Autodesk Fusion 360 part; units mm, degrees
note: some values were not read from the file. Set by a fixed rule: which face or edge a step refers to.
(part 2 of 2)
  arc A109 (-60.8901, 219.4175) -> (-60.8901, 225.0825) centre (-63.7145, 222.25) ccw construction
  line L110 (-63.3611, 192.0464) -> (-60.8901, 189.5825) construction
  arc A110 (-60.8901, 183.9175) -> (-60.8901, 189.5825) centre (-63.7145, 186.75) ccw construction
  line L111 (-60.8901, 183.9175) -> (-63.3611, 181.4536) construction
  arc A111 (-70.1855, 184.2861) -> (-63.3611, 181.4536) centre (-66.1855, 184.2861) ccw construction
  line L112 (-70.1855, 184.2861) -> (-70.1855, 189.2139) construction
  arc A112 (-63.3611, 192.0464) -> (-70.1855, 189.2139) centre (-66.1855, 189.2139) ccw construction
  line L113 (-60.8901, 148.4175) -> (-63.3611, 145.9536) construction
  arc A113 (-70.1855, 148.7861) -> (-63.3611, 145.9536) centre (-66.1855, 148.7861) ccw construction
  line L114 (-70.1855, 148.7861) -> (-70.1855, 153.7139) construction
  arc A114 (-63.3611, 156.5464) -> (-70.1855, 153.7139) centre (-66.1855, 153.7139) ccw construction
  line L115 (-63.3611, 156.5464) -> (-60.8901, 154.0825) construction
  arc A115 (-60.8901, 148.4175) -> (-60.8901, 154.0825) centre (-63.7145, 151.25) ccw construction
  line L116 (-63.3611, 121.0464) -> (-60.8901, 118.5825) construction
  arc A116 (-60.8901, 112.9175) -> (-60.8901, 118.5825) centre (-63.7145, 115.75) ccw construction
  line L117 (-60.8901, 112.9175) -> (-63.3611, 110.4536) construction
  arc A117 (-70.1855, 113.2861) -> (-63.3611, 110.4536) centre (-66.1855, 113.2861) ccw construction
  line L118 (-70.1855, 113.2861) -> (-70.1855, 118.2139) construction
  arc A118 (-63.3611, 121.0464) -> (-70.1855, 118.2139) centre (-66.1855, 118.2139) ccw construction
  line L119 (-55.2089, 159.715) -> (-61.6799, 166.1675) construction
  arc A119 (-61.6799, 171.8325) -> (-61.6799, 166.1675) centre (-58.8555, 169) ccw construction
  line L120 (-61.6799, 171.8325) -> (-55.2089, 178.285) construction
  arc A120 (-49.5601, 178.285) -> (-55.2089, 178.285) centre (-52.3845, 175.4525) ccw construction
  line L121 (-49.5601, 178.285) -> (-43.0891, 171.8325) construction
  arc A121 (-43.0891, 166.1675) -> (-43.0891, 171.8325) centre (-45.9135, 169) ccw construction
  line L122 (-43.0891, 166.1675) -> (-49.5601, 159.715) construction
  arc A122 (-55.2089, 159.715) -> (-49.5601, 159.715) centre (-52.3845, 162.5475) ccw construction
  circle A123 centre (-52.3845, 115.75) radius 3 construction
  line L123 (-49.5601, 213.785) -> (-43.0891, 207.3325) construction
  arc A124 (-43.0891, 201.6675) -> (-43.0891, 207.3325) centre (-45.9135, 204.5) ccw construction
  line L124 (-43.0891, 201.6675) -> (-49.5601, 195.215) construction
  arc A125 (-55.2089, 195.215) -> (-49.5601, 195.215) centre (-52.3845, 198.0475) ccw construction
  line L125 (-55.2089, 195.215) -> (-61.6799, 201.6675) construction
  arc A126 (-61.6799, 207.3325) -> (-61.6799, 201.6675) centre (-58.8555, 204.5) ccw construction
  line L126 (-61.6799, 207.3325) -> (-55.2089, 213.785) construction
  arc A127 (-49.5601, 213.785) -> (-55.2089, 213.785) centre (-52.3845, 210.9525) ccw construction
  line L127 (-49.5601, 142.785) -> (-43.0891, 136.3325) construction
  arc A128 (-43.0891, 130.6675) -> (-43.0891, 136.3325) centre (-45.9135, 133.5) ccw construction
  line L128 (-43.0891, 130.6675) -> (-49.5601, 124.215) construction
  arc A129 (-55.2089, 124.215) -> (-49.5601, 124.215) centre (-52.3845, 127.0475) ccw construction
  line L129 (-55.2089, 124.215) -> (-61.6799, 130.6675) construction
  arc A130 (-61.6799, 136.3325) -> (-61.6799, 130.6675) centre (-58.8555, 133.5) ccw construction
  line L130 (-61.6799, 136.3325) -> (-55.2089, 142.785) construction
  arc A131 (-49.5601, 142.785) -> (-55.2089, 142.785) centre (-52.3845, 139.9525) ccw construction
  circle A132 centre (-52.3845, 222.25) radius 3 construction
  circle A133 centre (-52.3845, 151.25) radius 3 construction
  circle A134 centre (-52.3845, 186.75) radius 3 construction
  line L131 (-57.6684, 104.8325) -> (-55.2089, 107.285) construction
  arc A135 (-49.5601, 107.285) -> (-55.2089, 107.285) centre (-52.3845, 104.4525) ccw construction
  line L132 (-49.5601, 107.285) -> (-47.1006, 104.8325) construction
  arc A136 (-49.925, 98) -> (-47.1006, 104.8325) centre (-49.925, 102) ccw construction
  line L133 (-49.925, 98) -> (-54.844, 98) construction
  arc A137 (-57.6684, 104.8325) -> (-54.844, 98) centre (-54.844, 102) ccw construction
  line L134 (-52.3845, 151.25) -> (52.3845, 151.25) construction
  circle A138 centre (-10, 151.25) radius 3.5
  circle A139 centre (10, 151.25) radius 3.5
  line L135 (0, 222.25) -> (0, 115.75) construction
  dimension "d99" = 7
  dimension "d100" = 20
  constraint coincident A133.centre L134.start
  constraint coincident A48.centre L134.end
  constraint coincident L134 A138.centre
  constraint coincident L134 A139.centre
  constraint coincident A90.centre L135.start
  constraint coincident A91.centre L135.end
  constraint equal A138 A139
  constraint symmetric A138 A139 L135
  measures "d99" diameter of A138
  measures "d100" distance of A138.centre A139.centre
extrude "Extrude12" cut sketch "Sketch13" against normal up to surface (18 mm away) contours L56 A52 L57 A139 | L56 A52 L57 A139 | L74 L76 A72 A138 | L74 L76 A72 A138
extrude "Extrude13" add sketch "Sketch13" against normal up to surface (18 mm away) contours L56 L57 A53 L58 A54 A139 | L74 A70 L75 A71 L76 A138 | A84
sketch "Sketch14" plane through (174.5, 0, 0) normal (1, 0, 0) x (0, 0, -1)
  circle A0 centre (-26.5204, 133.5) radius 7.5
  circle A1 centre (26.5204, 204.5) radius 7.5
  circle A2 centre (-26.5204, 169) radius 7.5
  circle A3 centre (26.5204, 133.5) radius 7.5
  circle A4 centre (26.5204, 169) radius 7.5
  circle A5 centre (-26.5204, 204.5) radius 7.5
  line L0 (-70.1855, 184.2861) -> (-70.1855, 189.2139)
  arc A6 (-63.3611, 192.0464) -> (-70.1855, 189.2139) centre (-66.1855, 189.2139) ccw
  line L1 (-63.3611, 192.0464) -> (-60.8901, 189.5825)
  arc A7 (-60.8901, 183.9175) -> (-60.8901, 189.5825) centre (-63.7145, 186.75) ccw
  line L2 (-60.8901, 183.9175) -> (-63.3611, 181.4536)
  arc A8 (-70.1855, 184.2861) -> (-63.3611, 181.4536) centre (-66.1855, 184.2861) ccw
  line L3 (-70.1855, 219.7861) -> (-70.1855, 224.7139)
  arc A9 (-63.3611, 227.5464) -> (-70.1855, 224.7139) centre (-66.1855, 224.7139) ccw
  line L4 (-63.3611, 227.5464) -> (-60.8901, 225.0825)
  arc A10 (-60.8901, 219.4175) -> (-60.8901, 225.0825) centre (-63.7145, 222.25) ccw
  line L5 (-60.8901, 219.4175) -> (-63.3611, 216.9536)
  arc A11 (-70.1855, 219.7861) -> (-63.3611, 216.9536) centre (-66.1855, 219.7861) ccw
  line L6 (-64.5205, 240) -> (-83, 240)
  line L7 (-83, 240) -> (-83, 116)
  line L8 (-83, 116) -> (-92, 107)
  line L9 (-92, 107) -> (-92, 90)
  line L10 (-92, 90) -> (92, 90)
  line L11 (92, 90) -> (92, 107)
  line L12 (92, 107) -> (83, 116)
  line L13 (83, 116) -> (83, 240)
  line L14 (83, 240) -> (64.5205, 240)
  line L15 (64.5205, 240) -> (55.2089, 230.715)
  arc A12 (49.5601, 230.715) -> (55.2089, 230.715) centre (52.3845, 233.5475) ccw
  line L16 (49.5601, 230.715) -> (40.2485, 240)
  line L17 (40.2485, 240) -> (12.7923, 240)
  line L18 (12.7923, 240) -> (2.7628, 230.4203)
  arc A13 (-2.7628, 230.4203) -> (2.7628, 230.4203) centre (0, 233.3129) ccw
  line L19 (-2.7628, 230.4203) -> (-12.7923, 240)
  line L20 (-12.7923, 240) -> (-40.2485, 240)
  line L21 (-40.2485, 240) -> (-49.5601, 230.715)
  arc A14 (-55.2089, 230.715) -> (-49.5601, 230.715) centre (-52.3845, 233.5475) ccw
  line L22 (-55.2089, 230.715) -> (-64.5205, 240)
  line L23 (-34.5835, 224.7139) -> (-34.5835, 219.7861)
  arc A15 (-41.4079, 216.9536) -> (-34.5835, 219.7861) centre (-38.5835, 219.7861) ccw
  line L24 (-41.4079, 216.9536) -> (-43.8789, 219.4175)
  arc A16 (-43.8789, 225.0825) -> (-43.8789, 219.4175) centre (-41.0545, 222.25) ccw
  line L25 (-43.8789, 225.0825) -> (-41.4079, 227.5464)
  arc A17 (-34.5835, 224.7139) -> (-41.4079, 227.5464) centre (-38.5835, 224.7139) ccw
  line L26 (-34.5835, 189.2139) -> (-34.5835, 184.2861)
  arc A18 (-41.4079, 181.4536) -> (-34.5835, 184.2861) centre (-38.5835, 184.2861) ccw
  line L27 (-41.4079, 181.4536) -> (-43.8789, 183.9175)
  arc A19 (-43.8789, 189.5825) -> (-43.8789, 183.9175) centre (-41.0545, 186.75) ccw
  line L28 (-43.8789, 189.5825) -> (-41.4079, 192.0464)
  arc A20 (-34.5835, 189.2139) -> (-41.4079, 192.0464) centre (-38.5835, 189.2139) ccw
  line L29 (-34.5835, 153.7139) -> (-34.5835, 148.7861)
  arc A21 (-41.4079, 145.9536) -> (-34.5835, 148.7861) centre (-38.5835, 148.7861) ccw
  line L30 (-41.4079, 145.9536) -> (-43.8789, 148.4175)
  arc A22 (-43.8789, 154.0825) -> (-43.8789, 148.4175) centre (-41.0545, 151.25) ccw
  line L31 (-43.8789, 154.0825) -> (-41.4079, 156.5464)
  arc A23 (-34.5835, 153.7139) -> (-41.4079, 156.5464) centre (-38.5835, 153.7139) ccw
  line L32 (-34.5835, 118.2139) -> (-34.5835, 113.2861)
  arc A24 (-41.4079, 110.4536) -> (-34.5835, 113.2861) centre (-38.5835, 113.2861) ccw
  line L33 (-41.4079, 110.4536) -> (-43.8789, 112.9175)
  arc A25 (-43.8789, 118.5825) -> (-43.8789, 112.9175) centre (-41.0545, 115.75) ccw
  line L34 (-43.8789, 118.5825) -> (-41.4079, 121.0464)
  arc A26 (-34.5835, 118.2139) -> (-41.4079, 121.0464) centre (-38.5835, 118.2139) ccw
  line L35 (-49.925, 98) -> (-54.844, 98)
  arc A27 (-57.6684, 104.8325) -> (-54.844, 98) centre (-54.844, 102) ccw
  line L36 (-57.6684, 104.8325) -> (-55.2089, 107.285)
  arc A28 (-49.5601, 107.285) -> (-55.2089, 107.285) centre (-52.3845, 104.4525) ccw
  line L37 (-49.5601, 107.285) -> (-47.1006, 104.8325)
  arc A29 (-49.925, 98) -> (-47.1006, 104.8325) centre (-49.925, 102) ccw
  line L38 (-70.1855, 113.2861) -> (-70.1855, 118.2139)
  arc A30 (-63.3611, 121.0464) -> (-70.1855, 118.2139) centre (-66.1855, 118.2139) ccw
  line L39 (-63.3611, 121.0464) -> (-60.8901, 118.5825)
  arc A31 (-60.8901, 112.9175) -> (-60.8901, 118.5825) centre (-63.7145, 115.75) ccw
  line L40 (-60.8901, 112.9175) -> (-63.3611, 110.4536)
  arc A32 (-70.1855, 113.2861) -> (-63.3611, 110.4536) centre (-66.1855, 113.2861) ccw
  circle A33 centre (-52.3845, 151.25) radius 3
  circle A34 centre (-52.3845, 115.75) radius 3
  line L41 (-61.6799, 207.3325) -> (-55.2089, 213.785)
  arc A35 (-49.5601, 213.785) -> (-55.2089, 213.785) centre (-52.3845, 210.9525) ccw
  line L42 (-49.5601, 213.785) -> (-43.0891, 207.3325)
  arc A36 (-43.0891, 201.6675) -> (-43.0891, 207.3325) centre (-45.9135, 204.5) ccw
  line L43 (-43.0891, 201.6675) -> (-49.5601, 195.215)
  arc A37 (-55.2089, 195.215) -> (-49.5601, 195.215) centre (-52.3845, 198.0475) ccw
  line L44 (-55.2089, 195.215) -> (-61.6799, 201.6675)
  arc A38 (-61.6799, 207.3325) -> (-61.6799, 201.6675) centre (-58.8555, 204.5) ccw
  line L45 (-43.0891, 166.1675) -> (-49.5601, 159.715)
  arc A39 (-55.2089, 159.715) -> (-49.5601, 159.715) centre (-52.3845, 162.5475) ccw
  line L46 (-55.2089, 159.715) -> (-61.6799, 166.1675)
  arc A40 (-61.6799, 171.8325) -> (-61.6799, 166.1675) centre (-58.8555, 169) ccw
  line L47 (-61.6799, 171.8325) -> (-55.2089, 178.285)
  arc A41 (-49.5601, 178.285) -> (-55.2089, 178.285) centre (-52.3845, 175.4525) ccw
  line L48 (-49.5601, 178.285) -> (-43.0891, 171.8325)
  arc A42 (-43.0891, 166.1675) -> (-43.0891, 171.8325) centre (-45.9135, 169) ccw
  circle A43 centre (-52.3845, 186.75) radius 3
  line L49 (-61.6799, 136.3325) -> (-55.2089, 142.785)
  arc A44 (-49.5601, 142.785) -> (-55.2089, 142.785) centre (-52.3845, 139.9525) ccw
  line L50 (-49.5601, 142.785) -> (-43.0891, 136.3325)
  arc A45 (-43.0891, 130.6675) -> (-43.0891, 136.3325) centre (-45.9135, 133.5) ccw
  line L51 (-43.0891, 130.6675) -> (-49.5601, 124.215)
  arc A46 (-55.2089, 124.215) -> (-49.5601, 124.215) centre (-52.3845, 127.0475) ccw
  line L52 (-55.2089, 124.215) -> (-61.6799, 130.6675)
  arc A47 (-61.6799, 136.3325) -> (-61.6799, 130.6675) centre (-58.8555, 133.5) ccw
  circle A48 centre (-52.3845, 222.25) radius 3
  circle A49 centre (-10, 151.25) radius 3.5
  line L53 (-18.5835, 183.8835) -> (-18.5835, 189.6165)
  arc A50 (-11.8207, 192.5091) -> (-18.5835, 189.6165) centre (-14.5835, 189.6165) ccw
  line L54 (-11.8207, 192.5091) -> (-8.8196, 189.6426)
  arc A51 (-8.8196, 183.8574) -> (-8.8196, 189.6426) centre (-11.5824, 186.75) ccw
  line L55 (-8.8196, 183.8574) -> (-11.8207, 180.9909)
  arc A52 (-18.5835, 183.8835) -> (-11.8207, 180.9909) centre (-14.5835, 183.8835) ccw
  line L56 (-18.5835, 219.3835) -> (-18.5835, 225.1165)
  arc A53 (-11.8207, 228.0091) -> (-18.5835, 225.1165) centre (-14.5835, 225.1165) ccw
  line L57 (-11.8207, 228.0091) -> (-8.8196, 225.1426)
  arc A54 (-8.8196, 219.3574) -> (-8.8196, 225.1426) centre (-11.5824, 222.25) ccw
  line L58 (-8.8196, 219.3574) -> (-11.8207, 216.4909)
  arc A55 (-18.5835, 219.3835) -> (-11.8207, 216.4909) centre (-14.5835, 219.3835) ccw
  line L59 (-60.8901, 148.4175) -> (-63.3611, 145.9536)
  arc A56 (-70.1855, 148.7861) -> (-63.3611, 145.9536) centre (-66.1855, 148.7861) ccw
  line L60 (-70.1855, 148.7861) -> (-70.1855, 153.7139)
  arc A57 (-63.3611, 156.5464) -> (-70.1855, 153.7139) centre (-66.1855, 153.7139) ccw
  line L61 (-63.3611, 156.5464) -> (-60.8901, 154.0825)
  arc A58 (-60.8901, 148.4175) -> (-60.8901, 154.0825) centre (-63.7145, 151.25) ccw
  line L62 (18.5835, 225.1165) -> (18.5835, 219.3835)
  arc A59 (11.8207, 216.4909) -> (18.5835, 219.3835) centre (14.5835, 219.3835) ccw
  line L63 (11.8207, 216.4909) -> (8.8196, 219.3574)
  arc A60 (8.8196, 225.1426) -> (8.8196, 219.3574) centre (11.5824, 222.25) ccw
  line L64 (8.8196, 225.1426) -> (11.8207, 228.0091)
  arc A61 (18.5835, 225.1165) -> (11.8207, 228.0091) centre (14.5835, 225.1165) ccw
  line L65 (18.5835, 189.6165) -> (18.5835, 183.8835)
  arc A62 (11.8207, 180.9909) -> (18.5835, 183.8835) centre (14.5835, 183.8835) ccw
  line L66 (11.8207, 180.9909) -> (8.8196, 183.8574)
  arc A63 (8.8196, 189.6426) -> (8.8196, 183.8574) centre (11.5824, 186.75) ccw
  line L67 (8.8196, 189.6426) -> (11.8207, 192.5091)
  arc A64 (18.5835, 189.6165) -> (11.8207, 192.5091) centre (14.5835, 189.6165) ccw
  circle A65 centre (10, 151.25) radius 3.5
  line L68 (18.5835, 118.6165) -> (18.5835, 112.8835)
  arc A66 (11.8207, 109.9909) -> (18.5835, 112.8835) centre (14.5835, 112.8835) ccw
  line L69 (11.8207, 109.9909) -> (8.8196, 112.8574)
  arc A67 (8.8196, 118.6426) -> (8.8196, 112.8574) centre (11.5824, 115.75) ccw
  line L70 (8.8196, 118.6426) -> (11.8207, 121.5091)
  arc A68 (18.5835, 118.6165) -> (11.8207, 121.5091) centre (14.5835, 118.6165) ccw
  line L71 (2.8133, 98) -> (-2.8133, 98)
  arc A69 (-5.5761, 104.8926) -> (-2.8133, 98) centre (-2.8133, 102) ccw
  line L72 (-5.5761, 104.8926) -> (-2.7628, 107.5797)
  arc A70 (2.7628, 107.5797) -> (-2.7628, 107.5797) centre (0, 104.6871) ccw
  line L73 (2.7628, 107.5797) -> (5.5761, 104.8926)
  arc A71 (2.8133, 98) -> (5.5761, 104.8926) centre (2.8133, 102) ccw
  circle A72 centre (0, 115.75) radius 3
  circle A73 centre (0, 222.25) radius 3
  circle A74 centre (0, 186.75) radius 3
  line L74 (9.7639, 166.1074) -> (2.7628, 159.4203)
  arc A75 (-2.7628, 159.4203) -> (2.7628, 159.4203) centre (0, 162.3129) ccw
  line L75 (-2.7628, 159.4203) -> (-9.7639, 166.1074)
  arc A76 (-9.7639, 171.8926) -> (-9.7639, 166.1074) centre (-7.0011, 169) ccw
  line L76 (-9.7639, 171.8926) -> (-2.7628, 178.5797)
  arc A77 (2.7628, 178.5797) -> (-2.7628, 178.5797) centre (0, 175.6871) ccw
  line L77 (2.7628, 178.5797) -> (9.7639, 171.8926)
  arc A78 (9.7639, 166.1074) -> (9.7639, 171.8926) centre (7.0011, 169) ccw
  line L78 (-9.7639, 207.3926) -> (-2.7628, 214.0797)
  arc A79 (2.7628, 214.0797) -> (-2.7628, 214.0797) centre (0, 211.1871) ccw
  line L79 (2.7628, 214.0797) -> (9.7639, 207.3926)
  arc A80 (9.7639, 201.6074) -> (9.7639, 207.3926) centre (7.0011, 204.5) ccw
  line L80 (9.7639, 201.6074) -> (2.7628, 194.9203)
  arc A81 (-2.7628, 194.9203) -> (2.7628, 194.9203) centre (0, 197.8129) ccw
  line L81 (-2.7628, 194.9203) -> (-9.7639, 201.6074)
  arc A82 (-9.7639, 207.3926) -> (-9.7639, 201.6074) centre (-7.0011, 204.5) ccw
  line L82 (-9.7639, 136.3926) -> (-2.7628, 143.0797)
  arc A83 (2.7628, 143.0797) -> (-2.7628, 143.0797) centre (0, 140.1871) ccw
  line L83 (2.7628, 143.0797) -> (9.7639, 136.3926)
  arc A84 (9.7639, 130.6074) -> (9.7639, 136.3926) centre (7.0011, 133.5) ccw
  line L84 (9.7639, 130.6074) -> (2.7628, 123.9203)
  arc A85 (-2.7628, 123.9203) -> (2.7628, 123.9203) centre (0, 126.8129) ccw
  line L85 (-2.7628, 123.9203) -> (-9.7639, 130.6074)
  arc A86 (-9.7639, 136.3926) -> (-9.7639, 130.6074) centre (-7.0011, 133.5) ccw
  line L86 (34.5835, 148.7861) -> (34.5835, 153.7139)
  arc A87 (41.4079, 156.5464) -> (34.5835, 153.7139) centre (38.5835, 153.7139) ccw
  line L87 (41.4079, 156.5464) -> (43.8789, 154.0825)
  arc A88 (43.8789, 148.4175) -> (43.8789, 154.0825) centre (41.0545, 151.25) ccw
  line L88 (43.8789, 148.4175) -> (41.4079, 145.9536)
  arc A89 (34.5835, 148.7861) -> (41.4079, 145.9536) centre (38.5835, 148.7861) ccw
  line L89 (34.5835, 184.2861) -> (34.5835, 189.2139)
  arc A90 (41.4079, 192.0464) -> (34.5835, 189.2139) centre (38.5835, 189.2139) ccw
  line L90 (41.4079, 192.0464) -> (43.8789, 189.5825)
  arc A91 (43.8789, 183.9175) -> (43.8789, 189.5825) centre (41.0545, 186.75) ccw
  line L91 (43.8789, 183.9175) -> (41.4079, 181.4536)
  arc A92 (34.5835, 184.2861) -> (41.4079, 181.4536) centre (38.5835, 184.2861) ccw
  line L92 (34.5835, 219.7861) -> (34.5835, 224.7139)
  arc A93 (41.4079, 227.5464) -> (34.5835, 224.7139) centre (38.5835, 224.7139) ccw
  line L93 (41.4079, 227.5464) -> (43.8789, 225.0825)
  arc A94 (43.8789, 219.4175) -> (43.8789, 225.0825) centre (41.0545, 222.25) ccw
  line L94 (43.8789, 219.4175) -> (41.4079, 216.9536)
  arc A95 (34.5835, 219.7861) -> (41.4079, 216.9536) centre (38.5835, 219.7861) ccw
  line L95 (-8.8196, 112.8574) -> (-11.8207, 109.9909)
  arc A96 (-18.5835, 112.8835) -> (-11.8207, 109.9909) centre (-14.5835, 112.8835) ccw
  line L96 (-18.5835, 112.8835) -> (-18.5835, 118.6165)
  arc A97 (-11.8207, 121.5091) -> (-18.5835, 118.6165) centre (-14.5835, 118.6165) ccw
  line L97 (-11.8207, 121.5091) -> (-8.8196, 118.6426)
  arc A98 (-8.8196, 112.8574) -> (-8.8196, 118.6426) centre (-11.5824, 115.75) ccw
  line L98 (70.1855, 224.7139) -> (70.1855, 219.7861)
  arc A99 (63.3611, 216.9536) -> (70.1855, 219.7861) centre (66.1855, 219.7861) ccw
  line L99 (63.3611, 216.9536) -> (60.8901, 219.4175)
  arc A100 (60.8901, 225.0825) -> (60.8901, 219.4175) centre (63.7145, 222.25) ccw
  line L100 (60.8901, 225.0825) -> (63.3611, 227.5464)
  arc A101 (70.1855, 224.7139) -> (63.3611, 227.5464) centre (66.1855, 224.7139) ccw
  line L101 (70.1855, 189.2139) -> (70.1855, 184.2861)
  arc A102 (63.3611, 181.4536) -> (70.1855, 184.2861) centre (66.1855, 184.2861) ccw
  line L102 (63.3611, 181.4536) -> (60.8901, 183.9175)
  arc A103 (60.8901, 189.5825) -> (60.8901, 183.9175) centre (63.7145, 186.75) ccw
  line L103 (60.8901, 189.5825) -> (63.3611, 192.0464)
  arc A104 (70.1855, 189.2139) -> (63.3611, 192.0464) centre (66.1855, 189.2139) ccw
  line L104 (70.1855, 153.7139) -> (70.1855, 148.7861)
  arc A105 (63.3611, 145.9536) -> (70.1855, 148.7861) centre (66.1855, 148.7861) ccw
  line L105 (63.3611, 145.9536) -> (60.8901, 148.4175)
  arc A106 (60.8901, 154.0825) -> (60.8901, 148.4175) centre (63.7145, 151.25) ccw
  line L106 (60.8901, 154.0825) -> (63.3611, 156.5464)
  arc A107 (70.1855, 153.7139) -> (63.3611, 156.5464) centre (66.1855, 153.7139) ccw
  line L107 (70.1855, 118.2139) -> (70.1855, 113.2861)
  arc A108 (63.3611, 110.4536) -> (70.1855, 113.2861) centre (66.1855, 113.2861) ccw
  line L108 (63.3611, 110.4536) -> (60.8901, 112.9175)
  arc A109 (60.8901, 118.5825) -> (60.8901, 112.9175) centre (63.7145, 115.75) ccw
  line L109 (60.8901, 118.5825) -> (63.3611, 121.0464)
  arc A110 (70.1855, 118.2139) -> (63.3611, 121.0464) centre (66.1855, 118.2139) ccw
  line L110 (54.844, 98) -> (49.925, 98)
  arc A111 (47.1006, 104.8325) -> (49.925, 98) centre (49.925, 102) ccw
  line L111 (47.1006, 104.8325) -> (49.5601, 107.285)
  arc A112 (55.2089, 107.285) -> (49.5601, 107.285) centre (52.3845, 104.4525) ccw
  line L112 (55.2089, 107.285) -> (57.6684, 104.8325)
  arc A113 (54.844, 98) -> (57.6684, 104.8325) centre (54.844, 102) ccw
  circle A114 centre (52.3845, 186.75) radius 3
  circle A115 centre (52.3845, 151.25) radius 3
  circle A116 centre (52.3845, 222.25) radius 3
  line L113 (43.0891, 136.3325) -> (49.5601, 142.785)
  arc A117 (55.2089, 142.785) -> (49.5601, 142.785) centre (52.3845, 139.9525) ccw
  line L114 (55.2089, 142.785) -> (61.6799, 136.3325)
  arc A118 (61.6799, 130.6675) -> (61.6799, 136.3325) centre (58.8555, 133.5) ccw
  line L115 (61.6799, 130.6675) -> (55.2089, 124.215)
  arc A119 (49.5601, 124.215) -> (55.2089, 124.215) centre (52.3845, 127.0475) ccw
  line L116 (49.5601, 124.215) -> (43.0891, 130.6675)
  arc A120 (43.0891, 136.3325) -> (43.0891, 130.6675) centre (45.9135, 133.5) ccw
  line L117 (43.0891, 207.3325) -> (49.5601, 213.785)
  arc A121 (55.2089, 213.785) -> (49.5601, 213.785) centre (52.3845, 210.9525) ccw
  line L118 (55.2089, 213.785) -> (61.6799, 207.3325)
  arc A122 (61.6799, 201.6675) -> (61.6799, 207.3325) centre (58.8555, 204.5) ccw
  line L119 (61.6799, 201.6675) -> (55.2089, 195.215)
  arc A123 (49.5601, 195.215) -> (55.2089, 195.215) centre (52.3845, 198.0475) ccw
  line L120 (49.5601, 195.215) -> (43.0891, 201.6675)
  arc A124 (43.0891, 207.3325) -> (43.0891, 201.6675) centre (45.9135, 204.5) ccw
  circle A125 centre (52.3845, 115.75) radius 3
  line L121 (61.6799, 166.1675) -> (55.2089, 159.715)
  arc A126 (49.5601, 159.715) -> (55.2089, 159.715) centre (52.3845, 162.5475) ccw
  line L122 (49.5601, 159.715) -> (43.0891, 166.1675)
  arc A127 (43.0891, 171.8325) -> (43.0891, 166.1675) centre (45.9135, 169) ccw
  line L123 (43.0891, 171.8325) -> (49.5601, 178.285)
  arc A128 (55.2089, 178.285) -> (49.5601, 178.285) centre (52.3845, 175.4525) ccw
  line L124 (55.2089, 178.285) -> (61.6799, 171.8325)
  arc A129 (61.6799, 166.1675) -> (61.6799, 171.8325) centre (58.8555, 169) ccw
  line L125 (43.8789, 112.9175) -> (41.4079, 110.4536)
  arc A130 (34.5835, 113.2861) -> (41.4079, 110.4536) centre (38.5835, 113.2861) ccw
  line L126 (34.5835, 113.2861) -> (34.5835, 118.2139)
  arc A131 (41.4079, 121.0464) -> (34.5835, 118.2139) centre (38.5835, 118.2139) ccw
  line L127 (41.4079, 121.0464) -> (43.8789, 118.5825)
  arc A132 (43.8789, 112.9175) -> (43.8789, 118.5825) centre (41.0545, 115.75) ccw
  line L128 (-5.75, 153.7037) -> (-10, 156.1575)
  line L129 (-10, 156.1575) -> (-14.25, 153.7037)
  line L130 (-14.25, 153.7037) -> (-14.25, 148.7963)
  line L131 (-14.25, 148.7963) -> (-10, 146.3425)
  line L132 (-10, 146.3425) -> (-5.75, 148.7963)
  line L133 (-5.75, 148.7963) -> (-5.75, 153.7037)
  line L134 (14.25, 153.7037) -> (10, 156.1575)
  line L135 (10, 156.1575) -> (5.75, 153.7037)
  line L136 (5.75, 153.7037) -> (5.75, 148.7963)
  line L137 (5.75, 148.7963) -> (10, 146.3425)
  line L138 (10, 146.3425) -> (14.25, 148.7963)
  line L139 (14.25, 148.7963) -> (14.25, 153.7037)
  point P0 (-10, 151.25)
  point P1 (10, 151.25)
  dimension "d105" = 4.25
  dimension "d106" = 4.25
  constraint coincident P0 A49.centre
  constraint parallel L29 L130
  constraint coincident P1 A65.centre
  constraint parallel L86 L139
  measures "d105" distance of P0 L133
  measures "d106" distance of P1 L139
extrude "Extrude14" cut sketch "Sketch14" against normal blind 15 contours L128 L129 L130 L131 L132 L133 | L134 L135 L136 L137 L138 L139
sketch "Sketch17" plane through (156.5, 0, 0) normal (-1, 0, 0) x (0, 0, 1)
  circle A0 centre (-10, 151.25) radius 3.5
  circle A1 centre (10, 151.25) radius 3.5
  circle A2 centre (26.5204, 133.5) radius 7.5
  circle A3 centre (-26.5204, 204.5) radius 7.5
  circle A4 centre (26.5204, 169) radius 7.5
  circle A5 centre (-26.5204, 133.5) radius 7.5
  circle A6 centre (-26.5204, 169) radius 7.5
  circle A7 centre (26.5204, 204.5) radius 7.5
  line L0 (70.1855, 153.7139) -> (70.1855, 148.7861)
  arc A8 (63.3611, 145.9536) -> (70.1855, 148.7861) centre (66.1855, 148.7861) ccw
  line L1 (63.3611, 145.9536) -> (60.8901, 148.4175)
  arc A9 (60.8901, 154.0825) -> (60.8901, 148.4175) centre (63.7145, 151.25) ccw
  line L2 (60.8901, 154.0825) -> (63.3611, 156.5464)
  arc A10 (70.1855, 153.7139) -> (63.3611, 156.5464) centre (66.1855, 153.7139) ccw
  line L3 (63.3611, 181.4536) -> (60.8901, 183.9175)
  arc A11 (60.8901, 189.5825) -> (60.8901, 183.9175) centre (63.7145, 186.75) ccw
  line L4 (60.8901, 189.5825) -> (63.3611, 192.0464)
  arc A12 (70.1855, 189.2139) -> (63.3611, 192.0464) centre (66.1855, 189.2139) ccw
  line L5 (70.1855, 189.2139) -> (70.1855, 184.2861)
  arc A13 (63.3611, 181.4536) -> (70.1855, 184.2861) centre (66.1855, 184.2861) ccw
  arc A14 (60.8901, 225.0825) -> (60.8901, 219.4175) centre (63.7145, 222.25) ccw
  line L6 (60.8901, 225.0825) -> (63.3611, 227.5464)
  arc A15 (70.1855, 224.7139) -> (63.3611, 227.5464) centre (66.1855, 224.7139) ccw
  line L7 (70.1855, 224.7139) -> (70.1855, 219.7861)
  arc A16 (63.3611, 216.9536) -> (70.1855, 219.7861) centre (66.1855, 219.7861) ccw
  line L8 (63.3611, 216.9536) -> (60.8901, 219.4175)
  line L9 (83, 240) -> (64.5205, 240)
  line L10 (64.5205, 240) -> (55.2089, 230.715)
  arc A17 (49.5601, 230.715) -> (55.2089, 230.715) centre (52.3845, 233.5475) ccw
  line L11 (49.5601, 230.715) -> (40.2485, 240)
  line L12 (40.2485, 240) -> (12.7923, 240)
  line L13 (12.7923, 240) -> (2.7628, 230.4203)
  arc A18 (-2.7628, 230.4203) -> (2.7628, 230.4203) centre (0, 233.3129) ccw
  line L14 (-2.7628, 230.4203) -> (-12.7923, 240)
  line L15 (-12.7923, 240) -> (-40.2485, 240)
  line L16 (-40.2485, 240) -> (-49.5601, 230.715)
  arc A19 (-55.2089, 230.715) -> (-49.5601, 230.715) centre (-52.3845, 233.5475) ccw
  line L17 (-55.2089, 230.715) -> (-64.5205, 240)
  line L18 (-64.5205, 240) -> (-83, 240)
  line L19 (-83, 240) -> (-83, 116)
  line L20 (-83, 116) -> (-92, 107)
  line L21 (-92, 107) -> (-92, 90)
  line L22 (-92, 90) -> (92, 90)
  line L23 (92, 90) -> (92, 107)
  line L24 (92, 107) -> (83, 116)
  line L25 (83, 116) -> (83, 240)
  line L26 (41.4079, 227.5464) -> (43.8789, 225.0825)
  arc A20 (43.8789, 219.4175) -> (43.8789, 225.0825) centre (41.0545, 222.25) ccw
  line L27 (43.8789, 219.4175) -> (41.4079, 216.9536)
  arc A21 (34.5835, 219.7861) -> (41.4079, 216.9536) centre (38.5835, 219.7861) ccw
  line L28 (34.5835, 219.7861) -> (34.5835, 224.7139)
  arc A22 (41.4079, 227.5464) -> (34.5835, 224.7139) centre (38.5835, 224.7139) ccw
  line L29 (43.8789, 183.9175) -> (41.4079, 181.4536)
  arc A23 (34.5835, 184.2861) -> (41.4079, 181.4536) centre (38.5835, 184.2861) ccw
  line L30 (34.5835, 184.2861) -> (34.5835, 189.2139)
  arc A24 (41.4079, 192.0464) -> (34.5835, 189.2139) centre (38.5835, 189.2139) ccw
  line L31 (41.4079, 192.0464) -> (43.8789, 189.5825)
  arc A25 (43.8789, 183.9175) -> (43.8789, 189.5825) centre (41.0545, 186.75) ccw
  line L32 (41.4079, 156.5464) -> (43.8789, 154.0825)
  arc A26 (43.8789, 148.4175) -> (43.8789, 154.0825) centre (41.0545, 151.25) ccw
  line L33 (43.8789, 148.4175) -> (41.4079, 145.9536)
  arc A27 (34.5835, 148.7861) -> (41.4079, 145.9536) centre (38.5835, 148.7861) ccw
  line L34 (34.5835, 148.7861) -> (34.5835, 153.7139)
  arc A28 (41.4079, 156.5464) -> (34.5835, 153.7139) centre (38.5835, 153.7139) ccw
  line L35 (43.8789, 112.9175) -> (41.4079, 110.4536)
  arc A29 (34.5835, 113.2861) -> (41.4079, 110.4536) centre (38.5835, 113.2861) ccw
  line L36 (34.5835, 113.2861) -> (34.5835, 118.2139)
  arc A30 (41.4079, 121.0464) -> (34.5835, 118.2139) centre (38.5835, 118.2139) ccw
  line L37 (41.4079, 121.0464) -> (43.8789, 118.5825)
  arc A31 (43.8789, 112.9175) -> (43.8789, 118.5825) centre (41.0545, 115.75) ccw
  line L38 (54.844, 98) -> (49.925, 98)
  arc A32 (47.1006, 104.8325) -> (49.925, 98) centre (49.925, 102) ccw
  line L39 (47.1006, 104.8325) -> (49.5601, 107.285)
  arc A33 (55.2089, 107.285) -> (49.5601, 107.285) centre (52.3845, 104.4525) ccw
  line L40 (55.2089, 107.285) -> (57.6684, 104.8325)
  arc A34 (54.844, 98) -> (57.6684, 104.8325) centre (54.844, 102) ccw
  circle A35 centre (52.3845, 222.25) radius 3
  line L41 (55.2089, 142.785) -> (61.6799, 136.3325)
  arc A36 (61.6799, 130.6675) -> (61.6799, 136.3325) centre (58.8555, 133.5) ccw
  line L42 (61.6799, 130.6675) -> (55.2089, 124.215)
  arc A37 (49.5601, 124.215) -> (55.2089, 124.215) centre (52.3845, 127.0475) ccw
  line L43 (49.5601, 124.215) -> (43.0891, 130.6675)
  arc A38 (43.0891, 136.3325) -> (43.0891, 130.6675) centre (45.9135, 133.5) ccw
  line L44 (43.0891, 136.3325) -> (49.5601, 142.785)
  arc A39 (55.2089, 142.785) -> (49.5601, 142.785) centre (52.3845, 139.9525) ccw
  circle A40 centre (52.3845, 186.75) radius 3
  line L45 (49.5601, 159.715) -> (43.0891, 166.1675)
  arc A41 (43.0891, 171.8325) -> (43.0891, 166.1675) centre (45.9135, 169) ccw
  line L46 (43.0891, 171.8325) -> (49.5601, 178.285)
  arc A42 (55.2089, 178.285) -> (49.5601, 178.285) centre (52.3845, 175.4525) ccw
  line L47 (55.2089, 178.285) -> (61.6799, 171.8325)
  arc A43 (61.6799, 166.1675) -> (61.6799, 171.8325) centre (58.8555, 169) ccw
  line L48 (61.6799, 166.1675) -> (55.2089, 159.715)
  arc A44 (49.5601, 159.715) -> (55.2089, 159.715) centre (52.3845, 162.5475) ccw
  line L49 (55.2089, 213.785) -> (61.6799, 207.3325)
  arc A45 (61.6799, 201.6675) -> (61.6799, 207.3325) centre (58.8555, 204.5) ccw
  line L50 (61.6799, 201.6675) -> (55.2089, 195.215)
  arc A46 (49.5601, 195.215) -> (55.2089, 195.215) centre (52.3845, 198.0475) ccw
  line L51 (49.5601, 195.215) -> (43.0891, 201.6675)
  arc A47 (43.0891, 207.3325) -> (43.0891, 201.6675) centre (45.9135, 204.5) ccw
  line L52 (43.0891, 207.3325) -> (49.5601, 213.785)
  arc A48 (55.2089, 213.785) -> (49.5601, 213.785) centre (52.3845, 210.9525) ccw
  circle A49 centre (52.3845, 115.75) radius 3
  circle A50 centre (52.3845, 151.25) radius 3
  line L53 (18.5835, 118.6165) -> (18.5835, 112.8835)
  arc A51 (11.8207, 109.9909) -> (18.5835, 112.8835) centre (14.5835, 112.8835) ccw
  line L54 (11.8207, 109.9909) -> (8.8196, 112.8574)
  arc A52 (8.8196, 118.6426) -> (8.8196, 112.8574) centre (11.5824, 115.75) ccw
  line L55 (8.8196, 118.6426) -> (11.8207, 121.5091)
  arc A53 (18.5835, 118.6165) -> (11.8207, 121.5091) centre (14.5835, 118.6165) ccw
  arc A54 (8.8196, 189.6426) -> (8.8196, 183.8574) centre (11.5824, 186.75) ccw
  line L56 (8.8196, 189.6426) -> (11.8207, 192.5091)
  arc A55 (18.5835, 189.6165) -> (11.8207, 192.5091) centre (14.5835, 189.6165) ccw
  line L57 (18.5835, 189.6165) -> (18.5835, 183.8835)
  arc A56 (11.8207, 180.9909) -> (18.5835, 183.8835) centre (14.5835, 183.8835) ccw
  line L58 (11.8207, 180.9909) -> (8.8196, 183.8574)
  line L59 (11.8207, 216.4909) -> (8.8196, 219.3574)
  arc A57 (8.8196, 225.1426) -> (8.8196, 219.3574) centre (11.5824, 222.25) ccw
  line L60 (8.8196, 225.1426) -> (11.8207, 228.0091)
  arc A58 (18.5835, 225.1165) -> (11.8207, 228.0091) centre (14.5835, 225.1165) ccw
  line L61 (18.5835, 225.1165) -> (18.5835, 219.3835)
  arc A59 (11.8207, 216.4909) -> (18.5835, 219.3835) centre (14.5835, 219.3835) ccw
  line L62 (63.3611, 110.4536) -> (60.8901, 112.9175)
  arc A60 (60.8901, 118.5825) -> (60.8901, 112.9175) centre (63.7145, 115.75) ccw
  line L63 (60.8901, 118.5825) -> (63.3611, 121.0464)
  arc A61 (70.1855, 118.2139) -> (63.3611, 121.0464) centre (66.1855, 118.2139) ccw
  line L64 (70.1855, 118.2139) -> (70.1855, 113.2861)
  arc A62 (63.3611, 110.4536) -> (70.1855, 113.2861) centre (66.1855, 113.2861) ccw
  line L65 (-8.8196, 219.3574) -> (-11.8207, 216.4909)
  arc A63 (-18.5835, 219.3835) -> (-11.8207, 216.4909) centre (-14.5835, 219.3835) ccw
  line L66 (-18.5835, 219.3835) -> (-18.5835, 225.1165)
  arc A64 (-11.8207, 228.0091) -> (-18.5835, 225.1165) centre (-14.5835, 225.1165) ccw
  line L67 (-11.8207, 228.0091) -> (-8.8196, 225.1426)
  arc A65 (-8.8196, 219.3574) -> (-8.8196, 225.1426) centre (-11.5824, 222.25) ccw
  line L68 (-11.8207, 192.5091) -> (-8.8196, 189.6426)
  arc A66 (-8.8196, 183.8574) -> (-8.8196, 189.6426) centre (-11.5824, 186.75) ccw
  line L69 (-8.8196, 183.8574) -> (-11.8207, 180.9909)
  arc A67 (-18.5835, 183.8835) -> (-11.8207, 180.9909) centre (-14.5835, 183.8835) ccw
  line L70 (-18.5835, 183.8835) -> (-18.5835, 189.6165)
  arc A68 (-11.8207, 192.5091) -> (-18.5835, 189.6165) centre (-14.5835, 189.6165) ccw
  line L71 (-11.8207, 121.5091) -> (-8.8196, 118.6426)
  arc A69 (-8.8196, 112.8574) -> (-8.8196, 118.6426) centre (-11.5824, 115.75) ccw
  line L72 (-8.8196, 112.8574) -> (-11.8207, 109.9909)
  arc A70 (-18.5835, 112.8835) -> (-11.8207, 109.9909) centre (-14.5835, 112.8835) ccw
  line L73 (-18.5835, 112.8835) -> (-18.5835, 118.6165)
  arc A71 (-11.8207, 121.5091) -> (-18.5835, 118.6165) centre (-14.5835, 118.6165) ccw
  line L74 (2.7628, 143.0797) -> (9.7639, 136.3926)
  arc A72 (9.7639, 130.6074) -> (9.7639, 136.3926) centre (7.0011, 133.5) ccw
  line L75 (9.7639, 130.6074) -> (2.7628, 123.9203)
  arc A73 (-2.7628, 123.9203) -> (2.7628, 123.9203) centre (0, 126.8129) ccw
  line L76 (-2.7628, 123.9203) -> (-9.7639, 130.6074)
  arc A74 (-9.7639, 136.3926) -> (-9.7639, 130.6074) centre (-7.0011, 133.5) ccw
  line L77 (-9.7639, 136.3926) -> (-2.7628, 143.0797)
  arc A75 (2.7628, 143.0797) -> (-2.7628, 143.0797) centre (0, 140.1871) ccw
  line L78 (2.7628, 214.0797) -> (9.7639, 207.3926)
  arc A76 (9.7639, 201.6074) -> (9.7639, 207.3926) centre (7.0011, 204.5) ccw
  line L79 (9.7639, 201.6074) -> (2.7628, 194.9203)
  arc A77 (-2.7628, 194.9203) -> (2.7628, 194.9203) centre (0, 197.8129) ccw
  line L80 (-2.7628, 194.9203) -> (-9.7639, 201.6074)
  arc A78 (-9.7639, 207.3926) -> (-9.7639, 201.6074) centre (-7.0011, 204.5) ccw
  line L81 (-9.7639, 207.3926) -> (-2.7628, 214.0797)
  arc A79 (2.7628, 214.0797) -> (-2.7628, 214.0797) centre (0, 211.1871) ccw
  line L82 (-2.7628, 159.4203) -> (-9.7639, 166.1074)
  arc A80 (-9.7639, 171.8926) -> (-9.7639, 166.1074) centre (-7.0011, 169) ccw
  line L83 (-9.7639, 171.8926) -> (-2.7628, 178.5797)
  arc A81 (2.7628, 178.5797) -> (-2.7628, 178.5797) centre (0, 175.6871) ccw
  line L84 (2.7628, 178.5797) -> (9.7639, 171.8926)
  arc A82 (9.7639, 166.1074) -> (9.7639, 171.8926) centre (7.0011, 169) ccw
  line L85 (9.7639, 166.1074) -> (2.7628, 159.4203)
  arc A83 (-2.7628, 159.4203) -> (2.7628, 159.4203) centre (0, 162.3129) ccw
  circle A84 centre (0, 186.75) radius 3
  circle A85 centre (0, 222.25) radius 3
  circle A86 centre (0, 115.75) radius 3
  line L86 (-34.5835, 118.2139) -> (-34.5835, 113.2861)
  arc A87 (-41.4079, 110.4536) -> (-34.5835, 113.2861) centre (-38.5835, 113.2861) ccw
  line L87 (-41.4079, 110.4536) -> (-43.8789, 112.9175)
  arc A88 (-43.8789, 118.5825) -> (-43.8789, 112.9175) centre (-41.0545, 115.75) ccw
  line L88 (-43.8789, 118.5825) -> (-41.4079, 121.0464)
  arc A89 (-34.5835, 118.2139) -> (-41.4079, 121.0464) centre (-38.5835, 118.2139) ccw
  line L89 (-41.4079, 145.9536) -> (-43.8789, 148.4175)
  arc A90 (-43.8789, 154.0825) -> (-43.8789, 148.4175) centre (-41.0545, 151.25) ccw
  line L90 (-43.8789, 154.0825) -> (-41.4079, 156.5464)
  arc A91 (-34.5835, 153.7139) -> (-41.4079, 156.5464) centre (-38.5835, 153.7139) ccw
  line L91 (-34.5835, 153.7139) -> (-34.5835, 148.7861)
  arc A92 (-41.4079, 145.9536) -> (-34.5835, 148.7861) centre (-38.5835, 148.7861) ccw
  arc A93 (-43.8789, 189.5825) -> (-43.8789, 183.9175) centre (-41.0545, 186.75) ccw
  line L92 (-43.8789, 189.5825) -> (-41.4079, 192.0464)
  arc A94 (-34.5835, 189.2139) -> (-41.4079, 192.0464) centre (-38.5835, 189.2139) ccw
  line L93 (-34.5835, 189.2139) -> (-34.5835, 184.2861)
  arc A95 (-41.4079, 181.4536) -> (-34.5835, 184.2861) centre (-38.5835, 184.2861) ccw
  line L94 (-41.4079, 181.4536) -> (-43.8789, 183.9175)
  line L95 (-41.4079, 216.9536) -> (-43.8789, 219.4175)
  arc A96 (-43.8789, 225.0825) -> (-43.8789, 219.4175) centre (-41.0545, 222.25) ccw
  line L96 (-43.8789, 225.0825) -> (-41.4079, 227.5464)
  arc A97 (-34.5835, 224.7139) -> (-41.4079, 227.5464) centre (-38.5835, 224.7139) ccw
  line L97 (-34.5835, 224.7139) -> (-34.5835, 219.7861)
  arc A98 (-41.4079, 216.9536) -> (-34.5835, 219.7861) centre (-38.5835, 219.7861) ccw
  line L98 (-5.5761, 104.8926) -> (-2.7628, 107.5797)
  arc A99 (2.7628, 107.5797) -> (-2.7628, 107.5797) centre (0, 104.6871) ccw
  line L99 (2.7628, 107.5797) -> (5.5761, 104.8926)
  arc A100 (2.8133, 98) -> (5.5761, 104.8926) centre (2.8133, 102) ccw
  line L100 (2.8133, 98) -> (-2.8133, 98)
  arc A101 (-5.5761, 104.8926) -> (-2.8133, 98) centre (-2.8133, 102) ccw
  line L101 (-60.8901, 219.4175) -> (-63.3611, 216.9536)
  arc A102 (-70.1855, 219.7861) -> (-63.3611, 216.9536) centre (-66.1855, 219.7861) ccw
  line L102 (-70.1855, 219.7861) -> (-70.1855, 224.7139)
  arc A103 (-63.3611, 227.5464) -> (-70.1855, 224.7139) centre (-66.1855, 224.7139) ccw
  line L103 (-63.3611, 227.5464) -> (-60.8901, 225.0825)
  arc A104 (-60.8901, 219.4175) -> (-60.8901, 225.0825) centre (-63.7145, 222.25) ccw
  line L104 (-63.3611, 192.0464) -> (-60.8901, 189.5825)
  arc A105 (-60.8901, 183.9175) -> (-60.8901, 189.5825) centre (-63.7145, 186.75) ccw
  line L105 (-60.8901, 183.9175) -> (-63.3611, 181.4536)
  arc A106 (-70.1855, 184.2861) -> (-63.3611, 181.4536) centre (-66.1855, 184.2861) ccw
  line L106 (-70.1855, 184.2861) -> (-70.1855, 189.2139)
  arc A107 (-63.3611, 192.0464) -> (-70.1855, 189.2139) centre (-66.1855, 189.2139) ccw
  line L107 (-60.8901, 148.4175) -> (-63.3611, 145.9536)
  arc A108 (-70.1855, 148.7861) -> (-63.3611, 145.9536) centre (-66.1855, 148.7861) ccw
  line L108 (-70.1855, 148.7861) -> (-70.1855, 153.7139)
  arc A109 (-63.3611, 156.5464) -> (-70.1855, 153.7139) centre (-66.1855, 153.7139) ccw
  line L109 (-63.3611, 156.5464) -> (-60.8901, 154.0825)
  arc A110 (-60.8901, 148.4175) -> (-60.8901, 154.0825) centre (-63.7145, 151.25) ccw
  line L110 (-63.3611, 121.0464) -> (-60.8901, 118.5825)
  arc A111 (-60.8901, 112.9175) -> (-60.8901, 118.5825) centre (-63.7145, 115.75) ccw
  line L111 (-60.8901, 112.9175) -> (-63.3611, 110.4536)
  arc A112 (-70.1855, 113.2861) -> (-63.3611, 110.4536) centre (-66.1855, 113.2861) ccw
  line L112 (-70.1855, 113.2861) -> (-70.1855, 118.2139)
  arc A113 (-63.3611, 121.0464) -> (-70.1855, 118.2139) centre (-66.1855, 118.2139) ccw
  line L113 (-55.2089, 159.715) -> (-61.6799, 166.1675)
  arc A114 (-61.6799, 171.8325) -> (-61.6799, 166.1675) centre (-58.8555, 169) ccw
  line L114 (-61.6799, 171.8325) -> (-55.2089, 178.285)
  arc A115 (-49.5601, 178.285) -> (-55.2089, 178.285) centre (-52.3845, 175.4525) ccw
  line L115 (-49.5601, 178.285) -> (-43.0891, 171.8325)
  arc A116 (-43.0891, 166.1675) -> (-43.0891, 171.8325) centre (-45.9135, 169) ccw
  line L116 (-43.0891, 166.1675) -> (-49.5601, 159.715)
  arc A117 (-55.2089, 159.715) -> (-49.5601, 159.715) centre (-52.3845, 162.5475) ccw
  circle A118 centre (-52.3845, 115.75) radius 3
  line L117 (-49.5601, 213.785) -> (-43.0891, 207.3325)
  arc A119 (-43.0891, 201.6675) -> (-43.0891, 207.3325) centre (-45.9135, 204.5) ccw
  line L118 (-43.0891, 201.6675) -> (-49.5601, 195.215)
  arc A120 (-55.2089, 195.215) -> (-49.5601, 195.215) centre (-52.3845, 198.0475) ccw
  line L119 (-55.2089, 195.215) -> (-61.6799, 201.6675)
  arc A121 (-61.6799, 207.3325) -> (-61.6799, 201.6675) centre (-58.8555, 204.5) ccw
  line L120 (-61.6799, 207.3325) -> (-55.2089, 213.785)
  arc A122 (-49.5601, 213.785) -> (-55.2089, 213.785) centre (-52.3845, 210.9525) ccw
  line L121 (-49.5601, 142.785) -> (-43.0891, 136.3325)
  arc A123 (-43.0891, 130.6675) -> (-43.0891, 136.3325) centre (-45.9135, 133.5) ccw
  line L122 (-43.0891, 130.6675) -> (-49.5601, 124.215)
  arc A124 (-55.2089, 124.215) -> (-49.5601, 124.215) centre (-52.3845, 127.0475) ccw
  line L123 (-55.2089, 124.215) -> (-61.6799, 130.6675)
  arc A125 (-61.6799, 136.3325) -> (-61.6799, 130.6675) centre (-58.8555, 133.5) ccw
  line L124 (-61.6799, 136.3325) -> (-55.2089, 142.785)
  arc A126 (-49.5601, 142.785) -> (-55.2089, 142.785) centre (-52.3845, 139.9525) ccw
  circle A127 centre (-52.3845, 222.25) radius 3
  circle A128 centre (-52.3845, 151.25) radius 3
  circle A129 centre (-52.3845, 186.75) radius 3
  line L125 (-57.6684, 104.8325) -> (-55.2089, 107.285)
  arc A130 (-49.5601, 107.285) -> (-55.2089, 107.285) centre (-52.3845, 104.4525) ccw
  line L126 (-49.5601, 107.285) -> (-47.1006, 104.8325)
  arc A131 (-49.925, 98) -> (-47.1006, 104.8325) centre (-49.925, 102) ccw
  line L127 (-49.925, 98) -> (-54.844, 98)
  arc A132 (-57.6684, 104.8325) -> (-54.844, 98) centre (-54.844, 102) ccw
  line L128 (-73, 240) -> (-73, 90)
  line L129 (0, 222.25) -> (0, 115.75) construction
  line L130 (-26.5204, 133.5) -> (26.5204, 133.5) construction
  line L131 (73, 240) -> (73, 90)
  line L132 (-83, 116) -> (-83, 90)
  line L133 (83, 116) -> (83, 90)
  line L134 (73, 133.5) -> (83, 133.5)
  line L135 (-73, 133.5) -> (-83, 133.5)
  dimension "d111" = 10
  constraint coincident L18 L128.start
  constraint coincident L22 L128.end
  constraint perpendicular L22 L128
  constraint coincident A85.centre L129.start
  constraint coincident A86.centre L129.end
  constraint coincident A5.centre L130.start
  constraint coincident A2.centre L130.end
  constraint coincident L9 L131.start
  constraint coincident L22 L131.end
  constraint perpendicular L22 L131
  constraint symmetric L128 L129 L131
  constraint coincident L19.end L20.start
  constraint coincident L22 L132.end
  constraint perpendicular L22 L132
  constraint coincident L24.end L25.start
  constraint coincident L22 L133.end
  constraint perpendicular L22 L133
  constraint coincident L131 L134.start
  constraint coincident L25 L134.end
  constraint perpendicular L25 L134
  constraint coincident L128 L135.start
  constraint coincident L19 L135.end
  constraint perpendicular L19 L135
  constraint collinear L130 L135
  constraint collinear L130 L134
  measures "d111" distance of L19 L128
extrude "Extrude15" add sketch "Sketch17" along normal blind 8 contours L22 L25 L131 L133 L134 | L19 L22 L128 L132 L135
equation "d26_1 = 150 mm - 8 mm"
equation "d28_1 = -150 mm + 25 mm"
equation "d35_1 = -8 mm - 18 mm"
equation "d48_1 = -150.00 mm + 8 mm"
equation "d107 = -18.00 mm + 3 mm"
